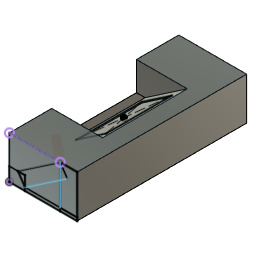
Second part (Autodesk Fusion 360 design; units mm, degrees)
Autodesk Fusion 360 part; units mm, degrees
sketch "Esquisse1" plane through (0, 0, 0) normal (0, 1, 0) x (1, 0, 0)
  line L0 (0, 0) -> (120, 0)
  line L1 (120, 0) -> (120, -100)
  line L2 (120, -100) -> (0, -100)
  line L3 (0, -100) -> (0, 0)
  line L4 (0, 0) -> (37.2, 0)
  line L5 (37.2, 0) -> (37.2, -32.2)
  line L6 (37.2, -32.2) -> (0, -32.2)
  line L7 (0, -32.2) -> (0, 0)
  line L8 (37.2, -32.2) -> (20.4, -32.2)
  line L9 (37.2, -7.4) -> (37.2, -32.2)
  line L10 (20.4, -32.2) -> (37.2, -7.4)
  line L11 (120, -100) -> (20.4, -32.2)
  line L12 (20.4, -32.2) -> (37.256, -7.4381)
  line L13 (37.256, -7.4381) -> (136.856, -75.2381)
  line L14 (136.856, -75.2381) -> (120, -100)
  line L15 (120, -100) -> (120, 0)
  line L16 (120, 0) -> (160, 0)
  line L17 (160, 0) -> (160, -100)
  line L18 (160, -100) -> (120, -100)
  line L19 (37.2, -7.4) -> (37.2, 0)
  line L20 (37.2, 0) -> (160, 0)
  line L21 (160, 0) -> (160, -7.4)
  line L22 (160, -7.4) -> (37.2, -7.4)
  line L23 (160, -7.4) -> (160, -100)
  line L24 (160, -100) -> (120, -100)
  line L25 (120, -100) -> (120, -7.4)
  line L26 (120, -7.4) -> (160, -7.4)
  dimension "d1" = 120
  dimension "d2" = 100
  dimension "d3" = 37.2
  dimension "d4" = 32.2
  dimension "d11" = 16.8
  dimension "d12" = 24.8
  dimension "d19" = 40
  constraint horizontal L0
  constraint vertical L1
  constraint horizontal L2
  constraint vertical L3
  constraint coincident L0.start L3.end
  constraint horizontal L4
  constraint vertical L5
  constraint horizontal L6
  constraint vertical L7
  constraint horizontal L8
  constraint vertical L9
  constraint perpendicular L11 L12
  constraint parallel L11 L13
  constraint parallel L12 L14
  constraint perpendicular L15 L16
  constraint parallel L15 L17
  constraint parallel L16 L18
  constraint perpendicular L19 L20
  constraint parallel L19 L21
  constraint parallel L20 L22
  constraint perpendicular L23 L24
  constraint parallel L23 L25
  constraint parallel L24 L26
  constraint perpendicular L22 L23
  measures "d1" distance of L0.start L0.end
  measures "d2" distance of L0.start L2.end
  measures "d3" distance of L0.start L4.end
  measures "d4" distance of L0.start L6.end
  measures "d11" distance of L5.end L8.end
  measures "d12" distance of L5.end L9.start
  measures "d19" distance of L1.end L17.end
extrude "Extrusion3" add sketch "Esquisse1" along normal blind 200 contours L0 L3 L4 L5 L6 L7 L10 L19 | L0 L1 L5 L15 L19 L20 L22 | L1 L15 L16 L17 L20 L21 L22 L26 | L5 L6 L8 L9 L12 | L1 L5 L6 L8 L9 L11 L12 L13 L15 L25 | L1 L13 L14 L15 L17 L18 L22 L23 L24 L25 L26 | L1 L13 L14 L15 L25
extrude "Extrusion4" add sketch "Esquisse1" along normal blind 100 contours L0 L1 L5 L15 L19 L20 L22 | L2 L3 L6 L11 | L1 L15 L16 L17 L20 L21 L22 L26 | L1 L5 L9 L12 L13 L15 L22 L25 | L1 L13 L14 L15 L17 L18 L22 L23 L24 L25 L26
mirror "Symétrie miroir2" about plane through (0, 200, 0) normal (0, 1, 0) of bodies 1 merged
sketch "Esquisse3" plane through (-8.5188, 0, 12.5143) normal (-0.562719, 0, 0.826649) x (0, -1, 0)
  line L0 (-100, 34.9832) -> (-100, 155.4697)
  line L1 (-100, 155.4697) -> (-300, 155.4697)
  line L2 (-300, 155.4697) -> (-300, 34.9832)
  line L3 (-300, 34.9832) -> (-100, 34.9832)
  line L4 (-277.5, 138.4697) -> (-122.5, 138.4697)
  line L5 (-122.5, 138.4697) -> (-122.5, 52.4697)
  line L6 (-122.5, 52.4697) -> (-277.5, 52.4697)
  line L7 (-277.5, 52.4697) -> (-277.5, 138.4697)
  line L8 (-277.5, 138.4697) -> (-122.5, 52.4697) construction
  line L9 (-122.5, 138.4697) -> (-277.5, 52.4697) construction
  point P0 (-200, 95.4697)
  dimension "d22" = 155
  dimension "d23" = 86
  dimension "d24" = 22.5
  dimension "d25" = 17
  constraint horizontal L4
  constraint perpendicular L4 L5
  constraint parallel L4 L6
  constraint parallel L5 L7
  constraint coincident L8 P0
  constraint coincident L9 P0
  measures "d22" distance of L5.end L6.end
  measures "d23" distance of L4.end L5.end
  measures "d24" distance of L2 L7
  measures "d25" distance of L1 L4
extrude "Extrusion6" cut sketch "Esquisse3" against normal blind 2 contours L4 L5 L6 L7
sketch "Esquisse4" plane through (0, 0, 100) normal (0, 0, 1) x (-1, 0, 0)
  line L0 (-160, 0) -> (-160, -400)
  line L1 (-160, -400) -> (0, -400)
  line L2 (0, -400) -> (0, -300)
  line L3 (0, -300) -> (-120, -300)
  line L4 (-120, -300) -> (-120, -100)
  line L5 (-120, -100) -> (0, -100)
  line L6 (0, -100) -> (0, 0)
  line L7 (0, 0) -> (-160, 0)
  line L8 (-120, -300) -> (-120, -400)
  dimension "d28" = 120
  dimension "d29" = 100
  dimension "d30" = 40
  constraint coincident L3.end L4.start
  constraint coincident L1 L8.end
  constraint perpendicular L1 L8
  measures "d28" distance of L2 L8
  measures "d29" distance of L1 L3
  measures "d30" distance of L0 L8
sketch "Esquisse5" plane through (0, 0, 100) normal (0, 0, 1) x (-1, 0, 0)
  line L0 (-160, 0) -> (-160, -400)
  line L1 (-160, -400) -> (0, -400)
  line L2 (0, -400) -> (0, -300)
  line L3 (0, -300) -> (-120, -300)
  line L4 (-120, -300) -> (-120, -100)
  line L5 (-120, -100) -> (0, -100)
  line L6 (0, -100) -> (0, 0)
  line L7 (0, 0) -> (-160, 0)
  line L8 (-120, 0) -> (0, 0)
  dimension "d31" = 400
  measures "d31" distance of L1 L8
